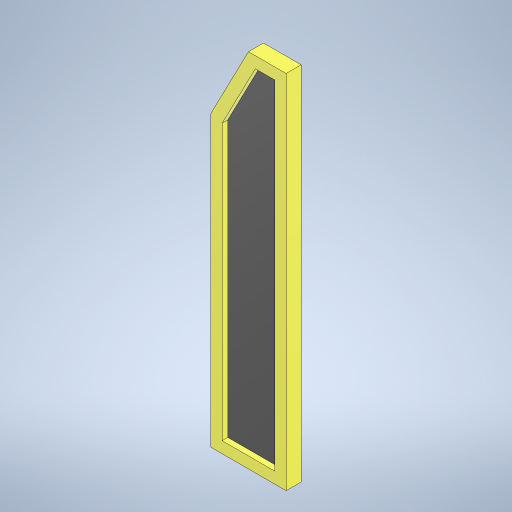
# Autodesk Inventor part: Side Plate
Saved by Autodesk Inventor 2023.2 (Build 272271000, 271)
## iProperties
Created: 2024-03-02
Part Number: Side Plate
Material: UHMW, White
Document SubType Name: Modeling
Designer: Nathan Cai
Mass: 27.4374 g
Surface Area: 114.558 cm^2
Volume: 29.1887 cm^3
Density: 0.94 g/cm^3
Appearance: Smooth - Yellow
Author: Nathan Cai
Autodesk Inventor part; units mm, degrees
ref_plane "YZ Plane" through (0, 0, 0) normal (1, 0, 0) x (0, 1, 0)
ref_plane "XZ Plane" through (0, 0, 0) normal (0, 1, 0) x (-1, 0, 0)
ref_plane "XY Plane" through (0, 0, 0) normal (0, 0, 1) x (1, 0, 0)
sketch "Sketch1" plane through (0, 0, 0) normal (0, 0, 1) x (1, 0, 0)
  line L0 (-15.875, -76.2) -> (15.875, -76.2)
  line L1 (15.875, -76.2) -> (15.875, 76.2)
  line L2 (15.875, 76.2) -> (-15.875, 76.2)
  line L3 (-15.875, 76.2) -> (-15.875, -76.2)
  line L4 (-15.875, -76.2) -> (15.875, 76.2) construction
  line L5 (15.875, -76.2) -> (-15.875, 76.2) construction
  line L6 (0, 76.2) -> (-15.875, 45.7044)
  point P0 (0, 0)
  dimension "d0" = 31.75
  dimension "d1" = 152.4
  dimension "d4" = 27.5
  dimension "d5" = 15.875
  constraints: 14 end point, 3 midpoint, 2 parallel, 1 horizontal, 1 perpendicular, 1 point on line
  measures "d0" distance of L2.end L1.end
  measures "d1" distance of L1.end L0.end
  measures "d4" angle of L1 L6
  measures "d5" distance from line of L1 L6.start
extrude "Extrusion1" add sketch "Sketch1" along normal blind 6.35 contours L3 L6 L2 L1 L0
sketch "Sketch2" plane through (0, 0, 6.35) normal (0, 0, 1) x (1, 0, 0)
  line L0 (15.875, 76.2) -> (0, 76.2) projected
  line L1 (0, 76.2) -> (-15.875, 45.7044) projected
  line L2 (-15.875, 45.7044) -> (-15.875, -76.2) projected
  line L3 (-15.875, -76.2) -> (15.875, -76.2) projected
  line L4 (15.875, -76.2) -> (15.875, 76.2) projected
  line L5 (-11.1125, -71.4375) -> (-11.1125, 44.539)
  line L6 (-11.1125, 44.539) -> (2.89, 71.4375)
  line L7 (2.89, 71.4375) -> (11.1125, 71.4375)
  line L8 (11.1125, 71.4375) -> (11.1125, -71.4375)
  line L9 (11.1125, -71.4375) -> (-11.1125, -71.4375)
  point P0 (0, 0)
  dimension "d6" = 4.7625
  constraints: 10 end point, 4 other
  measures "d6" distance between parallel lines of L2 L5
extrude "Extrusion2" cut sketch "Sketch2" against normal blind 2.3813 contours L5 L6 L7 L8 L9
sketch "Sketch3" plane through (0, 0, 0) normal (0, 0, -1) x (-1, 0, 0)
  line L0 (-15.875, 76.2) -> (0, 76.2) projected
  line L1 (-15.875, -76.2) -> (-15.875, 76.2) projected
  line L2 (15.875, -76.2) -> (-15.875, -76.2) projected
  line L3 (15.875, 45.7044) -> (15.875, -76.2) projected
  line L4 (0, 76.2) -> (15.875, 45.7044) projected
  line L5 (11.1125, -71.4375) -> (-11.1125, -71.4375)
  line L6 (-11.1125, -71.4375) -> (-11.1125, 71.4375)
  line L7 (-11.1125, 71.4375) -> (-2.89, 71.4375)
  line L8 (-2.89, 71.4375) -> (11.1125, 44.539)
  line L9 (11.1125, 44.539) -> (11.1125, -71.4375)
  point P0 (0, 0)
  dimension "d9" = 4.7625
  constraints: 10 end point, 4 other
  measures "d9" distance between parallel lines of L3 L9
extrude "Extrusion3" cut sketch "Sketch3" against normal blind 2.3813 contours L5 L6 L7 L8 L9
body "Solid1"
